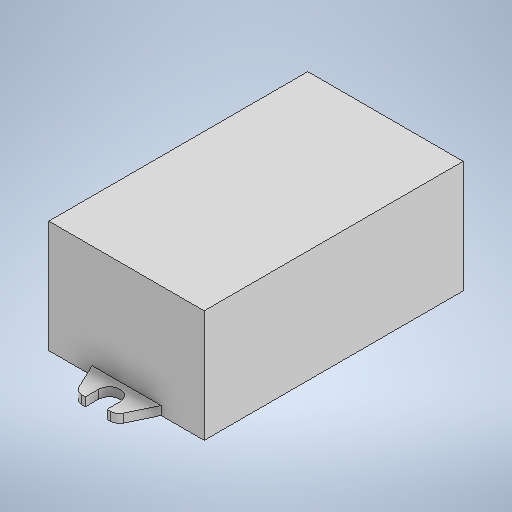
# Autodesk Inventor part: DC_DC_POWER
Saved by Autodesk Inventor 2025.4 (Build 294407000, 407)
## iProperties
Created: 2026-08-10
Part Number: DC_DC_POWER
Material: 常规
Document SubType Name: Modeling
Designer: Admin
Density: 1 g/cm^3
Appearance: 默认
Author: Admin
Autodesk Inventor part; units mm, degrees
ref_plane "YZ Plane" through (0, 0, 0) normal (1, 0, 0) x (0, 1, 0)
ref_plane "XZ Plane" through (0, 0, 0) normal (0, 1, 0) x (-1, 0, 0)
ref_plane "XY Plane" through (0, 0, 0) normal (0, 0, 1) x (1, 0, 0)
sketch "草图1" plane through (0, 0, 0) normal (0, 0, 1) x (1, 0, 0)
  line L0 (-18, -13) -> (18, -13)
  line L1 (18, -13) -> (18, 13)
  line L2 (18, 13) -> (-18, 13)
  line L3 (-18, 13) -> (-18, -13)
  point P0 (0, 0)
  point P1 (0, 13)
  point P2 (-18, 0)
  dimension "d0" = 36
  dimension "d1" = 26
  constraints: 8 end point, 2 midpoint, 2 parallel, 1 horizontal, 1 horizontal alignment, 1 perpendicular, 1 vertical alignment
  measures "d0" distance of L1.end L2.end
  measures "d1" distance of L2.end L0.start
extrude "拉伸1" add sketch "草图1" along normal mid plane 60
sketch "草图2" plane through (-18, -13, -30) normal (0, -1, 0) x (1, 0, 0)
  line L0 (0, 0) -> (0, 60) projected
  line L1 (36, 60) -> (0, 60) projected
  line L2 (36, 0) -> (0, 0) projected
  arc A0 (20.5, -4) -> (18, -1.5) centre (18, -4) ccw
  line L3 (21.3793, -7) -> (20.5, -7)
  line L4 (20.5, -7) -> (20.5, -4)
  line L5 (23.1821, -5.866) -> (26, 0)
  arc A1 (18, -1.5) -> (15.5, -4) centre (18, -4) ccw
  line L6 (14.6207, -7) -> (15.5, -7)
  line L7 (15.5, -7) -> (15.5, -4)
  line L8 (12.8179, -5.866) -> (10, 0)
  arc A2 (21.3793, -7) -> (23.1821, -5.866) centre (21.3793, -5) ccw
  arc A3 (12.8179, -5.866) -> (14.6207, -7) centre (14.6207, -5) ccw
  point P0 (18, 30)
  point P1 (22.6373, 30)
  point P2 (0, 30)
  point P3 (18, 0)
  point P4 (18, 30)
  point P5 (0, 30)
  point P6 (18, 0)
  point P7 (10, 0)
  dimension "d6" = 5
  dimension "d9" = 2
  constraints: 12 end point, 8 point on circle, 5 tangent, 4 centre point, 2 horizontal alignment, 2 midpoint, 1 equal radius, 1 horizontal, 1 vertical, 1 vertical alignment, 4 other
  measures "d6" diameter of A0
  measures "d9" radius of A2
extrude "拉伸2" add sketch "草图2" against normal blind 2
mirror "镜像1" about plane through (0, 0, 0) normal (0, 0, 1) of "拉伸2"
